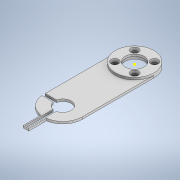
# Autodesk Inventor part: Pièce_moteur_maintient_test_3
Saved by Autodesk Inventor 2020.1 (Build 241239000, 239)
## iProperties
Created: 2019-07-26
Part Number: Pièce_moteur_maintient_test_3
Material: Générique
Document SubType Name: Modeling
Designer: marlo
Density: 1 g/cm^3
Appearance: Par défaut
Author: marlo
Autodesk Inventor part; units mm, degrees
ref_plane "YZ Plane" through (0, 0, 0) normal (1, 0, 0) x (0, 1, 0)
ref_plane "XZ Plane" through (0, 0, 0) normal (0, 1, 0) x (-1, 0, 0)
ref_plane "XY Plane" through (0, 0, 0) normal (0, 0, 1) x (1, 0, 0)
sketch "Esquisse3" plane through (0, 0, 0) normal (0, 1, 0) x (-1, 0, 0)
  line L0 (-6.5, 6.5) -> (6.5, 6.5) construction
  line L1 (6.5, 6.5) -> (6.5, -6.5) construction
  line L2 (6.5, -6.5) -> (-6.5, -6.5) construction
  line L3 (-6.5, -6.5) -> (-6.5, 6.5) construction
  line L4 (-6.5, 6.5) -> (6.5, -6.5) construction
  line L5 (6.5, 6.5) -> (-6.5, -6.5) construction
  line L6 (-11.5, 11.5) -> (11.5, 11.5) construction
  line L7 (11.5, 11.5) -> (11.5, -11.5) construction
  line L8 (11.5, -11.5) -> (-11.5, -11.5) construction
  line L9 (-11.5, -11.5) -> (-11.5, 11.5) construction
  line L10 (-11.5, 11.5) -> (11.5, -11.5) construction
  line L11 (11.5, 11.5) -> (-11.5, -11.5) construction
  line L12 (-6.5, 6.5) -> (-11.5, 6.5) construction
  line L13 (-11.5, 6.5) -> (-11.5, 11.5) construction
  line L14 (-11.5, 11.5) -> (-6.5, 11.5) construction
  line L15 (-6.5, 11.5) -> (-6.5, 6.5) construction
  line L16 (-6.5, -6.5) -> (-11.5, -6.5) construction
  line L17 (-11.5, -6.5) -> (-11.5, -11.5) construction
  line L18 (-11.5, -11.5) -> (-6.5, -11.5) construction
  line L19 (-6.5, -11.5) -> (-6.5, -6.5) construction
  line L20 (6.5, -6.5) -> (11.5, -6.5) construction
  line L21 (11.5, -6.5) -> (11.5, -11.5) construction
  line L22 (11.5, -11.5) -> (6.5, -11.5) construction
  line L23 (6.5, -11.5) -> (6.5, -6.5) construction
  line L24 (11.5, 11.5) -> (6.5, 11.5) construction
  line L25 (6.5, 11.5) -> (6.5, 6.5) construction
  line L26 (6.5, 6.5) -> (11.5, 6.5) construction
  line L27 (11.5, 6.5) -> (11.5, 11.5) construction
  circle A0 centre (9, 9) radius 2.5
  circle A1 centre (9, -9) radius 2.5
  circle A2 centre (-9, -9) radius 2.5
  circle A3 centre (-9, 9) radius 2.5
  circle A4 centre (0, 0) radius 17.5
  circle A5 centre (0, 0) radius 8.5
  line L28 (17.5, 0) -> (17.5, 65)
  line L29 (-17.5, 0) -> (-17.5, 65)
  line L30 (0, -17.5) -> (0, 82.5) construction
  circle A6 centre (0, 65) radius 17.5
  circle A7 centre (0, 65) radius 7.5
  line L31 (1.5, 72.3485) -> (-1.5, 72.3485)
  line L32 (-1.5, 72.3485) -> (-1.5, 97.3485)
  line L33 (-1.5, 97.3485) -> (1.5, 97.3485)
  line L34 (1.5, 97.3485) -> (1.5, 72.3485)
  line L35 (-2.5, 98.3485) -> (-2.5, 71.3485)
  line L36 (-2.5, 71.3485) -> (2.5, 71.3485)
  line L37 (2.5, 71.3485) -> (2.5, 98.3485)
  line L38 (2.5, 98.3485) -> (-2.5, 98.3485)
  line L39 (17.5, 63.5) -> (7.3485, 63.5)
  line L40 (7.3485, 63.5) -> (7.3485, 66.5)
  line L41 (7.3485, 66.5) -> (17.5, 66.5)
  line L42 (17.5, 66.5) -> (17.5, 63.5)
  point P0 (17.4356, 66.5)
  point P1 (2.5, 82.3205)
  point P2 (-2.5, 82.3205)
  dimension "d1" = 13
  dimension "d2" = 13
  dimension "d3" = 5
  dimension "d4" = 35
  dimension "d9" = 9
  dimension "d29" = 100
  dimension "d31" = 35
  dimension "d32" = 15
  dimension "d33" = 3
  dimension "d34" = 25
  dimension "d36" = 1
  dimension "d37" = 3
  constraints: 86 end point, 18 parallel, 13 tangent, 10 point on circle, 9 perpendicular, 8 centre point, 8 horizontal, 6 coincident, 3 point on line, 3 vertical, 2 midpoint, 3 other
  measures "d1" distance of L0.end L1.end
  measures "d2" distance of L0.start L0.end
  measures "d3" distance between parallel lines of L2 L8
  measures "d4" diameter of A4
  measures "d9" radial gap between concentric circles of A4 A5
  measures "d29" distance of L30.start L30.end
  measures "d31" diameter of A6
  measures "d32" diameter of A7
  measures "d33" distance of L32.end L33.end
  measures "d34" distance of L33.end L31.start
  measures "d36" distance between parallel lines of L32 L35
  measures "d37" distance of L41.end L39.start
extrude "Extrusion1" add sketch "Esquisse3" along normal blind 2 contours A4 | A4 L29 A6 L39 L28 | A6 L35 A7 L39 | L35 L38 L37 A6 L34 L33 L32 | A6 L32 A7 L35 | L41 A7 L37 A6 | L37 A7 L34 A6
sketch "Esquisse4" plane through (0, 2, 0) normal (0, 1, 0) x (-1, 0, 0)
  circle A0 centre (9, -9) radius 3.5
  circle A1 centre (9, -9) radius 2.5 projected
  circle A2 centre (-9, -9) radius 3.5
  circle A3 centre (-9, 9) radius 3.5
  circle A4 centre (9, 9) radius 3.5
  circle A5 centre (-9, -9) radius 2.5 projected
  circle A6 centre (-9, 9) radius 2.5 projected
  circle A7 centre (9, 9) radius 2.5 projected
  circle A8 centre (0, 0) radius 17.5
  circle A9 centre (0, 0) radius 8.544
  circle A10 centre (-9, -9) radius 2.5 projected
  circle A11 centre (-9, -9) radius 2.5
  circle A12 centre (-9, 9) radius 2.5
  circle A13 centre (9, 9) radius 2.5
  dimension "d10" = 7
  dimension "d11" = 7
  dimension "d12" = 7
  dimension "d13" = 7
  constraints: 9 centre point, 5 coincident, 4 concentric
  measures "d10" diameter of A0
  measures "d11" diameter of A2
  measures "d12" diameter of A3
  measures "d13" diameter of A4
extrude "Extrusion2" add sketch "Esquisse4" along normal blind 2 contours A0 | A2 | A3 | A4 | A8
chamfer "Chanfrein1" distance 1 distance2 2 1 edges at (-6.5, 4, -9) measured on face at (-3.3085, 4, -12.0053)
chamfer "Chanfrein2" distance 1 distance2 2 1 edges at (11.5, 4, -9) measured on face at (3.3085, 4, 12.0053)
chamfer "Chanfrein3" distance 1 distance2 2 1 edges at (-6.5, 4, 9) measured on face at (3.3085, 4, 12.0053)
chamfer "Chanfrein4" distance 1 distance2 2 1 edges at (11.5, 4, 9) measured on face at (3.3085, 4, 12.0053)
sketch "Esquisse7" plane through (0, 2, 0) normal (0, 1, 0) x (1, 0, 0)
  point P0 (0, 0)
